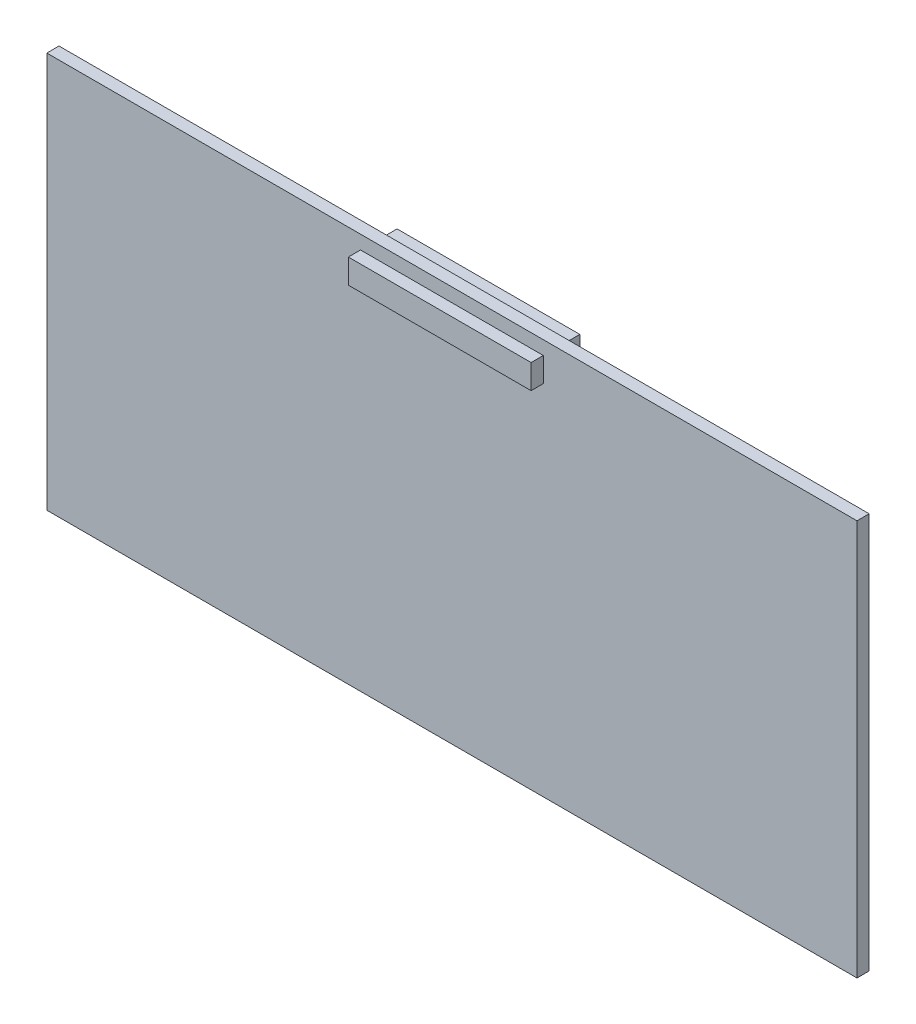
# Autodesk Inventor part: Top
Saved by Autodesk Inventor 2017 (Build 210142000, 142)
## iProperties
Created: 2016-12-08
Part Number: Top
Material: Generic
Document SubType Name: Modeling
Designer: SDL
Density: 1 g/cm^3
Appearance: Default
Author: SDL
Autodesk Inventor part; units mm, degrees
ref_plane "YZ Plane" through (0, 0, 0) normal (1, 0, 0) x (0, 1, 0)
ref_plane "XZ Plane" through (0, 0, 0) normal (0, 1, 0) x (-1, 0, 0)
ref_plane "XY Plane" through (0, 0, 0) normal (0, 0, 1) x (1, 0, 0)
sketch "Sketch1" plane through (0, 0, 0) normal (0, 0, 1) x (1, 0, 0)
  line L0 (-15, 2) -> (15, 2)
  line L1 (15, 2) -> (15, -2)
  line L2 (15, -2) -> (-15, -2)
  line L3 (-15, -2) -> (-15, 2)
  line L4 (-15, 2) -> (15, -2) construction
  line L5 (15, 2) -> (-15, -2) construction
  point P0 (0, 0)
  dimension "d0" = 30
  dimension "d1" = 4
  constraints: 12 end point, 2 midpoint, 2 parallel, 1 horizontal, 1 perpendicular
  measures "d0" distance of L1.end L2.end
  measures "d1" distance of L0.end L1.end
extrude "Extrusion1" add sketch "Sketch1" along normal blind 8
sketch "Sketch2" plane through (0, 0, 8) normal (0, 0, 1) x (1, 0, 0)
  point P0 (0, 0)
ref_plane "Work Plane2" through (0, -28.25, 4) normal (0, 0, 1) x (1, 0, 0)
sketch "Sketch4" plane through (0, -28.25, 4) normal (0, 0, 1) x (1, 0, 0)
  line L0 (-66.5, 32.5) -> (66.5, 32.5)
  line L1 (66.5, 32.5) -> (66.5, -32.5)
  line L2 (66.5, -32.5) -> (-66.5, -32.5)
  line L3 (-66.5, -32.5) -> (-66.5, 32.5)
  line L4 (-66.5, 32.5) -> (66.5, -32.5) construction
  line L5 (66.5, 32.5) -> (-66.5, -32.5) construction
  line L6 (15, 26.25) -> (15, 30.25) projected
  point P0 (0, 28.25)
  point P1 (0, 0)
  dimension "d4" = 133
  dimension "d5" = 65
  constraints: 12 end point, 3 parallel, 2 midpoint, 1 horizontal, 1 perpendicular
  measures "d4" distance of L1.end L2.end
  measures "d5" distance of L0.end L1.end
extrude "Extrusion2" add sketch "Sketch4" along normal blind 2
body "Solid1"
